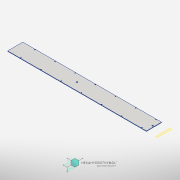
# Autodesk Inventor part: X-box-coverplate-2mm
Saved by Autodesk Inventor 2016 (Build 200138000, 138)
## iProperties
Created: 2015-04-22
Part Number: X-box-coverplate-2mm
Material: Aluminum 6061
Document SubType Name: Modeling
Designer: ax
Mass: 177.454 g
Surface Area: 684.903 cm^2
Volume: 65.7235 cm^3
Density: 2.7 g/cm^3
Appearance: Aluminum - Flat
Author: ax
Autodesk Inventor part; units mm, degrees
ref_plane "YZ Plane" through (0, 0, 0) normal (1, 0, 0) x (0, 1, 0)
ref_plane "XZ Plane" through (0, 0, 0) normal (0, 1, 0) x (-1, 0, 0)
ref_plane "XY Plane" through (0, 0, 0) normal (0, 0, 1) x (1, 0, 0)
ref_plane "Work Plane3" through (759.785, -2, 0) normal (0, 0, 1) x (-1, 0, 0)
sketch "Sketch2" plane through (759.785, -2, 0) normal (0, 0, 1) x (-1, 0, 0)
  line L0 (43.1075, -4) -> (593.1075, -4)
  line L1 (593.1075, -4) -> (593.1075, 56)
  line L2 (593.1075, 56) -> (43.1075, 56)
  line L3 (43.1075, 56) -> (43.1075, -4)
  point P0 (759.785, -2)
  dimension "d0" = 550
  dimension "d1" = 60
  constraints: 8 end point, 2 parallel, 1 horizontal, 1 perpendicular
  measures "d0" distance of L2.end L1.end
  measures "d1" distance of L1.end L0.end
extrude "Extrusion1" add sketch "Sketch2" along normal blind 2
sketch "Sketch4" plane through (759.785, -2, 2) normal (0, 0, 1) x (1, 0, 0)
  line L0 (-43.1075, 4) -> (-593.1075, 4) projected
  line L1 (-43.1075, -56) -> (-43.1075, 4) projected
  point P0 (-759.785, 2)
  point P1 (-48.1075, -26)
  point P2 (-348.1075, -26)
  point P3 (-648.1075, -26)
  dimension "d14" = 30
  dimension "d15" = 5
  dimension "d18" = 300
  constraints: 1 horizontal, 2 other
  measures "d14" distance from line of L0 point (-48.107, -26)
  measures "d15" distance from line of L1 point (-48.107, -26)
  measures "d18" distance of point (-48.107, -26) point (-348.107, -26)
hole "Hole2" at (111.6775, -28, 2) at (411.6775, -28, 2) at (711.6775, -28, 2) direction (0, 0, -1) diameter 5 end through all
chamfer "Chamfer1" [suppressed]
sketch "Sketch5" plane through (759.785, -2, 2) normal (0, 0, 1) x (1, 0, 0)
  line L0 (-43.1075, 4) -> (-593.1075, 4) projected
  line L1 (-43.1075, -56) -> (-43.1075, 4) projected
  point P0 (-63.1075, 1.5)
  point P1 (-143.1075, 1.5)
  point P2 (-223.1075, 1.5)
  point P3 (-303.1075, 1.5)
  point P4 (-383.1075, 1.5)
  point P5 (-463.1075, 1.5)
  point P6 (-543.1075, 1.5)
  point P7 (-63.1075, -53.5)
  point P8 (-143.1075, -53.5)
  point P9 (-223.1075, -53.5)
  point P10 (-303.1075, -53.5)
  point P11 (-383.1075, -53.5)
  point P12 (-463.1075, -53.5)
  point P13 (-543.1075, -53.5)
  dimension "d30" = 2.5
  dimension "d31" = 20
  dimension "d34" = 80
  dimension "d37" = 55
  constraints: 1 horizontal, 1 vertical, 13 other
  measures "d30" distance from line of L0 point (-63.107, 1.5)
  measures "d31" distance from line of L1 point (-63.107, 1.5)
  measures "d34" distance of point (-63.107, 1.5) point (-143.107, 1.5)
  measures "d37" distance of point (-63.107, 1.5) point (-63.107, -53.5)
hole "Hole3" at (536.6775, -55.5, 2) at (536.6775, -0.5, 2) at (456.6775, -0.5, 2) at (376.6775, -55.5, 2) at (376.6775, -0.5, 2) at (296.6775, -55.5, 2) at (296.6775, -0.5, 2) at (216.6775, -55.5, 2) at (216.6775, -0.5, 2) at (456.6775, -55.5, 2) at (696.6775, -55.5, 2) at (696.6775, -0.5, 2) at (616.6775, -55.5, 2) at (616.6775, -0.5, 2) direction (0, 0, -1) diameter 3 end through all
sketch "Sketch6" plane through (759.785, -2, 2) normal (0, 0, 1) x (1, 0, 0)
  line L0 (-415.5028, -23.6333) -> (-415.0497, -23.6333)
  line L1 (-415.0497, -23.6333) -> (-415.0497, -27.7161)
  line L2 (-415.0497, -27.7161) -> (-409.6296, -27.7161)
  line L3 (-409.6296, -27.7161) -> (-409.6296, -23.6333)
  line L4 (-409.6296, -23.6333) -> (-409.1821, -23.6333)
  line L5 (-409.1821, -23.6333) -> (-409.1821, -31.8699)
  line L6 (-409.1821, -31.8699) -> (-409.6296, -31.8699)
  line L7 (-409.6296, -31.8699) -> (-409.6296, -28.1582)
  line L8 (-409.6296, -28.1582) -> (-415.0497, -28.1582)
  line L9 (-415.0497, -28.1582) -> (-415.0497, -31.8699)
  line L10 (-415.0497, -31.8699) -> (-415.5028, -31.8699)
  line L11 (-415.5028, -31.8699) -> (-415.5028, -23.6333)
  line L12 (-423.5865, -23.5569) -> (-418.1391, -23.5569)
  line L13 (-418.1391, -23.5569) -> (-418.1391, -31.9518)
  line L14 (-418.1391, -31.9518) -> (-423.5865, -31.9518)
  line L15 (-423.5865, -31.9518) -> (-423.5865, -31.5151)
  line L16 (-423.5865, -31.5151) -> (-418.5867, -31.5151)
  line L17 (-418.5867, -31.5151) -> (-418.5867, -28.1582)
  line L18 (-418.5867, -28.1582) -> (-421.6324, -28.1582)
  line L19 (-421.6324, -28.1582) -> (-421.6324, -27.7161)
  line L20 (-421.6324, -27.7161) -> (-418.5867, -27.7161)
  line L21 (-418.5867, -27.7161) -> (-418.5867, -23.9827)
  line L22 (-418.5867, -23.9827) -> (-423.5865, -23.9827)
  line L23 (-423.5865, -23.9827) -> (-423.5865, -23.5569)
  line L24 (-431.5121, -23.7589) -> (-431.1136, -23.5624)
  line L25 (-431.1136, -23.5624) -> (-428.4991, -27.3504)
  line L26 (-428.4991, -27.3504) -> (-425.8791, -23.5569)
  line L27 (-425.8791, -23.5569) -> (-425.4861, -23.7589)
  line L28 (-425.4861, -23.7589) -> (-428.2207, -27.7434)
  line L29 (-428.2207, -27.7434) -> (-425.4916, -31.728)
  line L30 (-425.4916, -31.728) -> (-425.8791, -31.9572)
  line L31 (-425.8791, -31.9572) -> (-428.4991, -28.1474)
  line L32 (-428.4991, -28.1474) -> (-431.1136, -31.9572)
  line L33 (-431.1136, -31.9572) -> (-431.5121, -31.7335)
  line L34 (-431.5121, -31.7335) -> (-428.772, -27.7434)
  line L35 (-428.772, -27.7434) -> (-431.5121, -23.7589)
  line L36 (-440.0543, -23.7206) -> (-439.6504, -23.5733)
  line L37 (-439.6504, -23.5733) -> (-438.6023, -26.2041)
  line L38 (-438.6023, -26.2041) -> (-434.7434, -26.2041)
  line L39 (-434.7434, -26.2041) -> (-433.6953, -23.5733)
  line L40 (-433.6953, -23.5733) -> (-433.2914, -23.7206)
  line L41 (-433.2914, -23.7206) -> (-436.5228, -31.9518)
  line L42 (-436.5228, -31.9518) -> (-436.8284, -31.9518)
  line L43 (-436.8284, -31.9518) -> (-440.0543, -23.7206)
  line L44 (-438.4332, -26.6408) -> (-436.6756, -31.1221)
  line L45 (-436.6756, -31.1221) -> (-434.9125, -26.6408)
  line L46 (-434.9125, -26.6408) -> (-438.4332, -26.6408)
  line L47 (-448.2091, -23.6333) -> (-447.756, -23.6333)
  line L48 (-447.756, -23.6333) -> (-447.756, -27.7161)
  line L49 (-447.756, -27.7161) -> (-442.3359, -27.7161)
  line L50 (-442.3359, -27.7161) -> (-442.3359, -23.6333)
  line L51 (-442.3359, -23.6333) -> (-441.8884, -23.6333)
  line L52 (-441.8884, -23.6333) -> (-441.8884, -31.8699)
  line L53 (-441.8884, -31.8699) -> (-442.3359, -31.8699)
  line L54 (-442.3359, -31.8699) -> (-442.3359, -28.1582)
  line L55 (-442.3359, -28.1582) -> (-447.756, -28.1582)
  line L56 (-447.756, -28.1582) -> (-447.756, -31.8699)
  line L57 (-447.756, -31.8699) -> (-448.2091, -31.8699)
  line L58 (-448.2091, -31.8699) -> (-448.2091, -23.6333)
  line L59 (-457.5864, -31.6952) -> (-454.426, -27.8581)
  line L60 (-454.426, -27.8581) -> (-454.426, -23.6333)
  line L61 (-454.426, -23.6333) -> (-453.9729, -23.6333)
  line L62 (-453.9729, -23.6333) -> (-453.9729, -27.8581)
  line L63 (-453.9729, -27.8581) -> (-450.8181, -31.6952)
  line L64 (-450.8181, -31.6952) -> (-451.1566, -31.9791)
  line L65 (-451.1566, -31.9791) -> (-454.2023, -28.2893)
  line L66 (-454.2023, -28.2893) -> (-457.248, -31.9791)
  line L67 (-457.248, -31.9791) -> (-457.5864, -31.6952)
  line L68 (-464.5622, -26.7663) -> (-464.1473, -25.582)
  line L69 (-464.1473, -25.582) -> (-463.7489, -24.7686)
  line L70 (-463.7489, -24.7686) -> (-462.8865, -23.9499)
  line L71 (-462.8865, -23.9499) -> (-461.631, -23.5569)
  line L72 (-461.631, -23.5569) -> (-458.6344, -23.5569)
  line L73 (-458.6344, -23.5569) -> (-458.6344, -31.9518)
  line L74 (-458.6344, -31.9518) -> (-461.631, -31.9518)
  line L75 (-461.631, -31.9518) -> (-462.8865, -31.5425)
  line L76 (-462.8865, -31.5425) -> (-463.7489, -30.7291)
  line L77 (-463.7489, -30.7291) -> (-464.1473, -29.9158)
  line L78 (-464.1473, -29.9158) -> (-464.5622, -28.726)
  line L79 (-464.5622, -28.726) -> (-464.5622, -26.7663)
  line L80 (-464.1091, -26.832) -> (-464.1091, -28.6659)
  line L81 (-464.1091, -28.6659) -> (-463.7435, -29.7521)
  line L82 (-463.7435, -29.7521) -> (-463.3668, -30.4617)
  line L83 (-463.3668, -30.4617) -> (-462.6517, -31.1658)
  line L84 (-462.6517, -31.1658) -> (-461.5655, -31.5151)
  line L85 (-461.5655, -31.5151) -> (-459.082, -31.5151)
  line L86 (-459.082, -31.5151) -> (-459.082, -23.9827)
  line L87 (-459.082, -23.9827) -> (-461.5655, -23.9827)
  line L88 (-461.5655, -23.9827) -> (-462.6517, -24.3321)
  line L89 (-462.6517, -24.3321) -> (-463.3668, -25.0361)
  line L90 (-463.3668, -25.0361) -> (-463.7435, -25.7456)
  line L91 (-463.7435, -25.7456) -> (-464.1091, -26.832)
  line L92 (-472.7388, -29.4028) -> (-472.3075, -28.5622)
  line L93 (-472.3075, -28.5622) -> (-471.8436, -28.1256)
  line L94 (-471.8436, -28.1256) -> (-470.5882, -27.7161)
  line L95 (-470.5882, -27.7161) -> (-470.1952, -27.7161)
  line L96 (-470.1952, -27.7161) -> (-472.7878, -23.7589)
  line L97 (-472.7878, -23.7589) -> (-472.384, -23.5569)
  line L98 (-472.384, -23.5569) -> (-469.6548, -27.7161)
  line L99 (-469.6548, -27.7161) -> (-467.2586, -27.7161)
  line L100 (-467.2586, -27.7161) -> (-467.2586, -23.6333)
  line L101 (-467.2586, -23.6333) -> (-466.811, -23.6333)
  line L102 (-466.811, -23.6333) -> (-466.811, -31.9518)
  line L103 (-466.811, -31.9518) -> (-470.5882, -31.9518)
  line L104 (-470.5882, -31.9518) -> (-471.8436, -31.5425)
  line L105 (-471.8436, -31.5425) -> (-472.3075, -31.1112)
  line L106 (-472.3075, -31.1112) -> (-472.7388, -30.2652)
  line L107 (-472.7388, -30.2652) -> (-472.7388, -29.4028)
  line L108 (-472.2857, -29.512) -> (-472.2857, -30.1615)
  line L109 (-472.2857, -30.1615) -> (-471.9309, -30.8437)
  line L110 (-471.9309, -30.8437) -> (-471.6089, -31.1658)
  line L111 (-471.6089, -31.1658) -> (-470.5228, -31.5151)
  line L112 (-470.5228, -31.5151) -> (-467.2586, -31.5151)
  line L113 (-467.2586, -31.5151) -> (-467.2586, -28.1582)
  line L114 (-467.2586, -28.1582) -> (-470.5228, -28.1582)
  line L115 (-470.5228, -28.1582) -> (-471.6089, -28.5076)
  line L116 (-471.6089, -28.5076) -> (-471.9309, -28.8297)
  line L117 (-471.9309, -28.8297) -> (-472.2857, -29.512)
  line L118 (-481.3082, -26.7663) -> (-480.8934, -25.582)
  line L119 (-480.8934, -25.582) -> (-480.4895, -24.7686)
  line L120 (-480.4895, -24.7686) -> (-479.6544, -23.9609)
  line L121 (-479.6544, -23.9609) -> (-478.7865, -23.5569)
  line L122 (-478.7865, -23.5569) -> (-477.1107, -23.5569)
  line L123 (-477.1107, -23.5569) -> (-476.2484, -23.9609)
  line L124 (-476.2484, -23.9609) -> (-475.4079, -24.7686)
  line L125 (-475.4079, -24.7686) -> (-475.0093, -25.582)
  line L126 (-475.0093, -25.582) -> (-474.5946, -26.7663)
  line L127 (-474.5946, -26.7663) -> (-474.5946, -28.726)
  line L128 (-474.5946, -28.726) -> (-475.0093, -29.9158)
  line L129 (-475.0093, -29.9158) -> (-475.4079, -30.7291)
  line L130 (-475.4079, -30.7291) -> (-476.2484, -31.537)
  line L131 (-476.2484, -31.537) -> (-477.1107, -31.9518)
  line L132 (-477.1107, -31.9518) -> (-478.7865, -31.9518)
  line L133 (-478.7865, -31.9518) -> (-479.6544, -31.537)
  line L134 (-479.6544, -31.537) -> (-480.4895, -30.7291)
  line L135 (-480.4895, -30.7291) -> (-480.8934, -29.9158)
  line L136 (-480.8934, -29.9158) -> (-481.3082, -28.726)
  line L137 (-481.3082, -28.726) -> (-481.3082, -26.7663)
  line L138 (-480.8552, -26.832) -> (-480.8552, -28.6659)
  line L139 (-480.8552, -28.6659) -> (-480.484, -29.7521)
  line L140 (-480.484, -29.7521) -> (-480.1129, -30.4617)
  line L141 (-480.1129, -30.4617) -> (-479.376, -31.1713)
  line L142 (-479.376, -31.1713) -> (-478.6774, -31.5151)
  line L143 (-478.6774, -31.5151) -> (-477.2254, -31.5151)
  line L144 (-477.2254, -31.5151) -> (-476.5213, -31.1713)
  line L145 (-476.5213, -31.1713) -> (-475.7899, -30.4617)
  line L146 (-475.7899, -30.4617) -> (-475.4133, -29.7521)
  line L147 (-475.4133, -29.7521) -> (-475.0475, -28.6659)
  line L148 (-475.0475, -28.6659) -> (-475.0475, -26.832)
  line L149 (-475.0475, -26.832) -> (-475.4133, -25.7456)
  line L150 (-475.4133, -25.7456) -> (-475.7899, -25.0361)
  line L151 (-475.7899, -25.0361) -> (-476.5213, -24.3265)
  line L152 (-476.5213, -24.3265) -> (-477.2254, -23.9827)
  line L153 (-477.2254, -23.9827) -> (-478.6774, -23.9827)
  line L154 (-478.6774, -23.9827) -> (-479.376, -24.3265)
  line L155 (-479.376, -24.3265) -> (-480.1129, -25.0361)
  line L156 (-480.1129, -25.0361) -> (-480.484, -25.7456)
  line L157 (-480.484, -25.7456) -> (-480.8552, -26.832)
  line L158 (-489.3976, -31.5151) -> (-486.7449, -31.5151)
  line L159 (-486.7449, -31.5151) -> (-486.7449, -23.6333)
  line L160 (-486.7449, -23.6333) -> (-486.2918, -23.6333)
  line L161 (-486.2918, -23.6333) -> (-486.2918, -31.5151)
  line L162 (-486.2918, -31.5151) -> (-483.6445, -31.5151)
  line L163 (-483.6445, -31.5151) -> (-483.6445, -31.9518)
  line L164 (-483.6445, -31.9518) -> (-489.3976, -31.9518)
  line L165 (-489.3976, -31.9518) -> (-489.3976, -31.5151)
  line L166 (-496.8809, -23.6333) -> (-496.4278, -23.6333)
  line L167 (-496.4278, -23.6333) -> (-496.4278, -27.7161)
  line L168 (-496.4278, -27.7161) -> (-491.0077, -27.7161)
  line L169 (-491.0077, -27.7161) -> (-491.0077, -23.6333)
  line L170 (-491.0077, -23.6333) -> (-490.5601, -23.6333)
  line L171 (-490.5601, -23.6333) -> (-490.5601, -31.8699)
  line L172 (-490.5601, -31.8699) -> (-491.0077, -31.8699)
  line L173 (-491.0077, -31.8699) -> (-491.0077, -28.1582)
  line L174 (-491.0077, -28.1582) -> (-496.4278, -28.1582)
  line L175 (-496.4278, -28.1582) -> (-496.4278, -31.8699)
  line L176 (-496.4278, -31.8699) -> (-496.8809, -31.8699)
  line L177 (-496.8809, -31.8699) -> (-496.8809, -23.6333)
  line L178 (-506.2582, -31.6952) -> (-503.0978, -27.8581)
  line L179 (-503.0978, -27.8581) -> (-503.0978, -23.6333)
  line L180 (-503.0978, -23.6333) -> (-502.6449, -23.6333)
  line L181 (-502.6449, -23.6333) -> (-502.6449, -27.8581)
  line L182 (-502.6449, -27.8581) -> (-499.4899, -31.6952)
  line L183 (-499.4899, -31.6952) -> (-499.8283, -31.9791)
  line L184 (-499.8283, -31.9791) -> (-502.8741, -28.2893)
  line L185 (-502.8741, -28.2893) -> (-505.9198, -31.9791)
  line L186 (-505.9198, -31.9791) -> (-506.2582, -31.6952)
  line L187 (-514.0147, -23.6333) -> (-513.567, -23.6333)
  line L188 (-513.567, -23.6333) -> (-513.567, -30.549)
  line L189 (-513.567, -30.549) -> (-510.8489, -23.6333)
  line L190 (-510.8489, -23.6333) -> (-510.4777, -23.6333)
  line L191 (-510.4777, -23.6333) -> (-507.754, -30.549)
  line L192 (-507.754, -30.549) -> (-507.754, -23.6333)
  line L193 (-507.754, -23.6333) -> (-507.3063, -23.6333)
  line L194 (-507.3063, -23.6333) -> (-507.3063, -31.9518)
  line L195 (-507.3063, -31.9518) -> (-507.6831, -31.9518)
  line L196 (-507.6831, -31.9518) -> (-510.6633, -24.3701)
  line L197 (-510.6633, -24.3701) -> (-513.6381, -31.9518)
  line L198 (-513.6381, -31.9518) -> (-514.0147, -31.9518)
  line L199 (-514.0147, -31.9518) -> (-514.0147, -23.6333)
  line L200 (-522.9772, -26.7663) -> (-522.5624, -25.582)
  line L201 (-522.5624, -25.582) -> (-522.1585, -24.7686)
  line L202 (-522.1585, -24.7686) -> (-521.3234, -23.9609)
  line L203 (-521.3234, -23.9609) -> (-520.4555, -23.5569)
  line L204 (-520.4555, -23.5569) -> (-518.7797, -23.5569)
  line L205 (-518.7797, -23.5569) -> (-517.9173, -23.9609)
  line L206 (-517.9173, -23.9609) -> (-517.0768, -24.7686)
  line L207 (-517.0768, -24.7686) -> (-516.6782, -25.582)
  line L208 (-516.6782, -25.582) -> (-516.2635, -26.7663)
  line L209 (-516.2635, -26.7663) -> (-516.2635, -28.726)
  line L210 (-516.2635, -28.726) -> (-516.6782, -29.9158)
  line L211 (-516.6782, -29.9158) -> (-517.0768, -30.7291)
  line L212 (-517.0768, -30.7291) -> (-517.9173, -31.537)
  line L213 (-517.9173, -31.537) -> (-518.7797, -31.9518)
  line L214 (-518.7797, -31.9518) -> (-520.4555, -31.9518)
  line L215 (-520.4555, -31.9518) -> (-521.3234, -31.537)
  line L216 (-521.3234, -31.537) -> (-522.1585, -30.7291)
  line L217 (-522.1585, -30.7291) -> (-522.5624, -29.9158)
  line L218 (-522.5624, -29.9158) -> (-522.9772, -28.726)
  line L219 (-522.9772, -28.726) -> (-522.9772, -26.7663)
  line L220 (-522.5241, -26.832) -> (-522.5241, -28.6659)
  line L221 (-522.5241, -28.6659) -> (-522.1529, -29.7521)
  line L222 (-522.1529, -29.7521) -> (-521.7819, -30.4617)
  line L223 (-521.7819, -30.4617) -> (-521.0449, -31.1713)
  line L224 (-521.0449, -31.1713) -> (-520.3463, -31.5151)
  line L225 (-520.3463, -31.5151) -> (-518.8944, -31.5151)
  line L226 (-518.8944, -31.5151) -> (-518.1902, -31.1713)
  line L227 (-518.1902, -31.1713) -> (-517.4588, -30.4617)
  line L228 (-517.4588, -30.4617) -> (-517.0822, -29.7521)
  line L229 (-517.0822, -29.7521) -> (-516.7165, -28.6659)
  line L230 (-516.7165, -28.6659) -> (-516.7165, -26.832)
  line L231 (-516.7165, -26.832) -> (-517.0822, -25.7456)
  line L232 (-517.0822, -25.7456) -> (-517.4588, -25.0361)
  line L233 (-517.4588, -25.0361) -> (-518.1902, -24.3265)
  line L234 (-518.1902, -24.3265) -> (-518.8944, -23.9827)
  line L235 (-518.8944, -23.9827) -> (-520.3463, -23.9827)
  line L236 (-520.3463, -23.9827) -> (-521.0449, -24.3265)
  line L237 (-521.0449, -24.3265) -> (-521.7819, -25.0361)
  line L238 (-521.7819, -25.0361) -> (-522.1529, -25.7456)
  line L239 (-522.1529, -25.7456) -> (-522.5241, -26.832)
  line L240 (-529.8929, -23.5569) -> (-525.2259, -23.5569)
  line L241 (-525.2259, -23.5569) -> (-525.2259, -31.8699)
  line L242 (-525.2259, -31.8699) -> (-525.6735, -31.8699)
  line L243 (-525.6735, -31.8699) -> (-525.6735, -23.9827)
  line L244 (-525.6735, -23.9827) -> (-529.8929, -23.9827)
  line L245 (-529.8929, -23.9827) -> (-529.8929, -23.5569)
  line L246 (-533.4625, -30.8056) -> (-533.337, -30.4235)
  line L247 (-533.337, -30.4235) -> (-533.0205, -30.1232)
  line L248 (-533.0205, -30.1232) -> (-532.6329, -29.9977)
  line L249 (-532.6329, -29.9977) -> (-532.2781, -29.9977)
  line L250 (-532.2781, -29.9977) -> (-531.8906, -30.1232)
  line L251 (-531.8906, -30.1232) -> (-531.5739, -30.4235)
  line L252 (-531.5739, -30.4235) -> (-531.4484, -30.8056)
  line L253 (-531.4484, -30.8056) -> (-531.4484, -31.1494)
  line L254 (-531.4484, -31.1494) -> (-531.5739, -31.5206)
  line L255 (-531.5739, -31.5206) -> (-531.8851, -31.8317)
  line L256 (-531.8851, -31.8317) -> (-532.2781, -31.9518)
  line L257 (-532.2781, -31.9518) -> (-532.6329, -31.9518)
  line L258 (-532.6329, -31.9518) -> (-533.0259, -31.8317)
  line L259 (-533.0259, -31.8317) -> (-533.337, -31.5206)
  line L260 (-533.337, -31.5206) -> (-533.4625, -31.1494)
  line L261 (-533.4625, -31.1494) -> (-533.4625, -30.8056)
  line L262 (-533.0095, -30.8656) -> (-533.0095, -31.084)
  line L263 (-533.0095, -31.084) -> (-532.9386, -31.2804)
  line L264 (-532.9386, -31.2804) -> (-532.7694, -31.4442)
  line L265 (-532.7694, -31.4442) -> (-532.5674, -31.5151)
  line L266 (-532.5674, -31.5151) -> (-532.3436, -31.5151)
  line L267 (-532.3436, -31.5151) -> (-532.1417, -31.4442)
  line L268 (-532.1417, -31.4442) -> (-531.9725, -31.2804)
  line L269 (-531.9725, -31.2804) -> (-531.896, -31.084)
  line L270 (-531.896, -31.084) -> (-531.896, -30.871)
  line L271 (-531.896, -30.871) -> (-531.9725, -30.6691)
  line L272 (-531.9725, -30.6691) -> (-532.1417, -30.5054)
  line L273 (-532.1417, -30.5054) -> (-532.3436, -30.4344)
  line L274 (-532.3436, -30.4344) -> (-532.5674, -30.4344)
  line L275 (-532.5674, -30.4344) -> (-532.7694, -30.5054)
  line L276 (-532.7694, -30.5054) -> (-532.9386, -30.6691)
  line L277 (-532.9386, -30.6691) -> (-533.0095, -30.8656)
  line L278 (-403.6046, -22.2059) -> (-394.3046, -16.8672)
  line L279 (-394.3046, -16.8672) -> (-385.0046, -22.2059)
  line L280 (-385.0046, -22.2059) -> (-385.0046, -32.8835)
  line L281 (-385.0046, -32.8835) -> (-394.3046, -38.2223)
  line L282 (-394.3046, -38.2223) -> (-403.6046, -32.8835)
  line L283 (-403.6046, -32.8835) -> (-403.6046, -22.2059)
  line L284 (-413.0822, -38.2183) -> (-403.8372, -32.8795)
  line L285 (-385.3472, -32.8795) -> (-376.1022, -38.2183)
  line L286 (-385.3472, -22.2099) -> (-375.9019, -16.7555)
  line L287 (-375.9019, -16.7555) -> (-366.7571, -22.0324)
  line L288 (-375.9019, -6.1055) -> (-375.9019, -16.7555)
  point P0 (-759.785, 2)
  dimension "d3" = 0
  constraints: 578 end point
body "Solid1"
